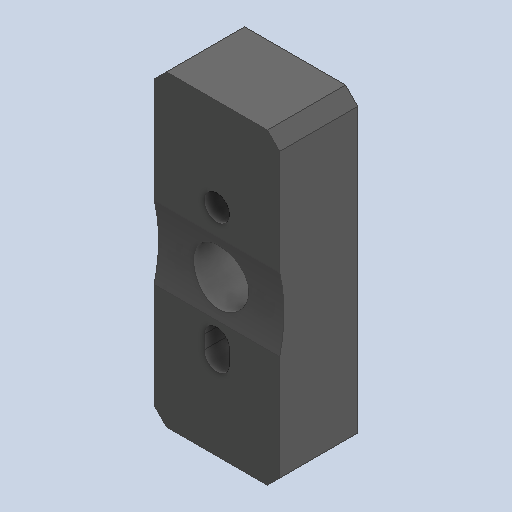
# Autodesk Inventor part: POLARIS-K05S1-adapter
Saved by Autodesk Inventor 2024.2 (Build 282272000, 272)
## iProperties
Created: 2021-02-18
Part Number: POLARIS-K05S1-adapter
Material: Generic
Document SubType Name: Modeling
Designer: maria
Density: 1 g/cm^3
Appearance: Default
Mass: 1.44702 g
Surface Area: 10.7533 cm^2
Volume: 1.44702 cm^3
ItemSpecifications: {"_id":"602eaaf1ef1d9f0009ff0b96","finish":"543ef1f380da5b0c476373c1","finish_location":null,"material":"5515e170db035c20ce34af9a","process_initialism":null,"quotes":null,"current_quote":null,"quantity_ordered":1,"features":null,"hardware":null,"threading":null,"part_markings":[],"surface_roughness":null,"tolerance":null,"weld_quantity":null,"Notes":"","certifications":[],"part":null,"revision_num":0,"last_history":null,"inspection_requirement_details":{"inspection_requirement":"std","customer_data_sheet":null},"feedback":null}
Author: maria
Autodesk Inventor part; units mm, degrees
ref_plane "YZ Plane" through (0, 0, 0) normal (1, 0, 0) x (0, 1, 0)
ref_plane "XZ Plane" through (0, 0, 0) normal (0, 1, 0) x (-1, 0, 0)
ref_plane "XY Plane" through (0, 0, 0) normal (0, 0, 1) x (1, 0, 0)
sketch "Sketch1" plane through (0, 0, 0) normal (0, 0, 1) x (1, 0, 0)
  line L0 (-10.2, -12.5) -> (0, -12.5)
  line L1 (0, -12.5) -> (0, 12.5)
  line L2 (0, 12.5) -> (-10.2, 12.5)
  line L3 (-10.2, 12.5) -> (-10.2, -12.5)
  point P0 (0, 0)
  dimension "MIRROR_WIDTH" = 10.2
  dimension "WIDTH" = 10.2
  dimension "LENGTH" = 25
  dimension "d3" = 12.5
  constraints: 8 end point, 2 parallel, 1 horizontal, 1 perpendicular
  measures "MIRROR_WIDTH" distance from line of L3 point (0, 0)
  measures "WIDTH" distance of L0.start L0.end
  measures "LENGTH" distance of L2.end L0.start
  measures "d3" distance from line of L2 point (0, 0)
extrude "Extrusion1" add sketch "Sketch1" along normal blind 6.35
sketch "Sketch2" plane through (0, 0, 6.35) normal (0, 0, 1) x (1, 0, 0)
  line L0 (0, 12.5) -> (2, 12.5)
  line L1 (2, 12.5) -> (2, -12.5)
  line L2 (2, -12.5) -> (0, -12.5)
  line L3 (0, -12.5) -> (0, 12.5)
  point P0 (0, 0)
  dimension "d6" = 2
  dimension "d7" = 25
  dimension "d8" = 12.5
  dimension "d9" = 0
  constraints: 8 end point, 2 parallel, 1 horizontal, 1 perpendicular
  measures "d6" distance of L0.start L0.end
  measures "d7" distance of L0.end L1.end
  measures "d8" distance from line of L0 point (0, 0)
  measures "d9" distance from line of point (0, 0) L3
extrude "Extrusion2" [suppressed]
sketch "Sketch3" plane through (0, 0, 6.35) normal (0, 0, 1) x (1, 0, 0)
  point P0 (0, 0)
  point P1 (-5.1, 0)
  dimension "d12" = 5.1
  dimension "d13" = 0
  measures "d12" distance of point (0, 0) point (-5.1, 0)
  measures "d13" vertical distance of point (0, 0) point (-5.1, 0)
hole "Hole1" at (-5.1, 0, 6.35) direction (0, 0, -1) diameter 4.5 depth 12.3 clearance for "Socket Head Cap Screw" size "#8" standard "Ansi Unified Screw Threads"
sketch "Sketch4" plane through (0, 0, 0) normal (0, 0, -1) x (-1, 0, 0)
  circle A0 centre (5.1, 0) radius 2.25 projected
  line L0 (5.1, -5.5455) -> (5.1, -4.4545) construction
  line L1 (6.15, -5.5455) -> (6.15, -4.4545)
  line L2 (4.05, -4.4545) -> (4.05, -5.5455)
  arc A1 (4.05, -5.5455) -> (6.15, -5.5455) centre (5.1, -5.5455) ccw
  arc A2 (6.15, -4.4545) -> (4.05, -4.4545) centre (5.1, -4.4545) ccw
  point P0 (0, 0)
  point P1 (5.1, -5)
  point P2 (5.1, 5)
  dimension "d21" = 0
  dimension "d22" = 0
  dimension "d23" = 5
  dimension "d24" = 5
  dimension "d43" = 1.05
  dimension "d44" = 1.091
  constraints: 8 end point, 4 point on circle, 4 tangent, 2 centre point, 1 midpoint, 1 parallel, 1 vertical
  measures "d21" horizontal distance of point (5.1, 5) point (5.1, -5)
  measures "d22" horizontal distance of A0.centre point (5.1, -5)
  measures "d23" distance of point (5.1, -5) A0.centre
  measures "d24" distance of point (5.1, 5) A0.centre
  measures "d43" radius of A2
  measures "d44" distance of L2.start L2.end
hole "Hole2" at (-5.1, 5, 0) direction (0, 0, 1) diameter 2.1 end through all
extrude "Extrusion3" cut sketch "Sketch4" against normal through all contours A1 L2 A2 L1
chamfer "Chamfer1" distance 1 angle 45 4 edges at (-10.2, -12.5, 3.175) (0, -12.5, 3.175) (0, 12.5, 3.175) (-10.2, 12.5, 3.175)
sketch "Sketch6" plane through (0, -11.5, 0) normal (1, 0, 0) x (0, 0, -1)
  circle A0 centre (-18.7, 11.5) radius 12.7
  point P0 (0, 11.5)
  dimension "d50" = 25.4
  dimension "d51" = 0
  dimension "d52" = 18.7
  constraints: 1 centre point
  measures "d50" diameter of A0
  measures "d51" vertical distance of point (0, 11.5) A0.centre
  measures "d52" distance of A0.centre point (0, 11.5)
extrude "Extrusion4" cut sketch "Sketch6" against normal up to surface (10.2 mm away)
equation "\"WIDTH\" = MIRROR_WIDTH"
equation "\"d3\" = 0.5 * LENGTH"
equation "\"d7\" = LENGTH"
equation "\"d8\" = 0.5 * LENGTH"
equation "\"d12\" = 0.5 * MIRROR_WIDTH"
equation "\"d24\" = d23"
body "Solid1"
